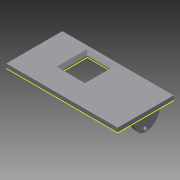
# Autodesk Inventor part: obudowa - timer- back
Saved by Autodesk Inventor 2014 (Build 180170000, 170)
## iProperties
Created: 2018-02-28
Part Number: obudowa - timer- back
Material: Generic
Document SubType Name: Modeling
Designer: HP820
Density: 1 g/cm^3
Appearance: Default
Author: HP820
Autodesk Inventor part; units mm, degrees
ref_plane "YZ Plane" through (0, 0, 0) normal (1, 0, 0) x (0, 1, 0)
ref_plane "XZ Plane" through (0, 0, 0) normal (0, 1, 0) x (-1, 0, 0)
ref_plane "XY Plane" through (0, 0, 0) normal (0, 0, 1) x (1, 0, 0)
sketch "Sketch1" plane through (0, 0, 0) normal (0, 0, 1) x (1, 0, 0)
  line L0 (40, 20.5) -> (40, -20.5) projected
  line L1 (-40, 20.5) -> (40, 20.5) projected
  line L2 (-40, -20.5) -> (-40, 20.5) projected
  line L3 (40, -20.5) -> (-40, -20.5) projected
  line L4 (40, 20.5) -> (40, -20.5) projected
  line L5 (40, -20.5) -> (-40, -20.5) projected
  line L6 (-40, -20.5) -> (-40, 20.5) projected
  line L7 (-40, 20.5) -> (40, 20.5) projected
  line L8 (37, 23.5) -> (-37, 23.5) projected
  line L9 (-43, 17.5) -> (-43, -17.5) projected
  line L10 (-37, -23.5) -> (37, -23.5) projected
  line L11 (43, -17.5) -> (43, 17.5) projected
  line L12 (34.23, -11.25) -> (34.23, 10.75) projected
  line L13 (5.23, -11.25) -> (34.23, -11.25) projected
  line L14 (5.23, 10.75) -> (5.23, -11.25) projected
  line L15 (34.23, 10.75) -> (5.23, 10.75) projected
  circle A0 centre (-26.5, 0.5) radius 5 projected
  arc A1 (37, -23.5) -> (43, -17.5) centre (37, -17.5) ccw projected
  arc A2 (43, 17.5) -> (37, 23.5) centre (37, 17.5) ccw projected
  arc A3 (-37, 23.5) -> (-43, 17.5) centre (-37, 17.5) ccw projected
  arc A4 (-43, -17.5) -> (-37, -23.5) centre (-37, -17.5) ccw projected
  point P0 (0, 0)
extrude "Extrusion1" add sketch "Sketch1" along normal blind 3 contours L0 L3 L2 L1 | A2 L11 A1 L10 A4 L9 A3 L8 | L13 L14 L15 L12 | A0
sketch "Sketch2" plane through (0, 0, 3) normal (0, 0, 1) x (1, 0, 0)
  line L0 (39.5, 20) -> (-39.5, 20) projected
  line L1 (-39.5, 20) -> (-39.5, -20) projected
  line L2 (-39.5, -20) -> (39.5, -20) projected
  line L3 (39.5, -20) -> (39.5, 20) projected
  line L4 (-17.5, 15.5) -> (-1.5, 15.5)
  line L5 (-1.5, 15.5) -> (-1.5, -2)
  line L6 (-1.5, -2) -> (-17.5, -2)
  line L7 (-17.5, -2) -> (-17.5, 15.5)
  line L8 (-17.5, 15.5) -> (-1.5, -2) construction
  line L9 (-1.5, 15.5) -> (-17.5, -2) construction
  point P0 (0, 0)
  point P1 (-9.5, 6.75)
  dimension "d2" = 16
  dimension "d3" = 17.5
  dimension "d4" = 18
  dimension "d6" = 41
  constraints: 12 end point, 2 midpoint, 2 parallel, 1 horizontal, 1 perpendicular
  measures "d2" distance of L5.end L6.end
  measures "d3" distance of L4.end L5.end
  measures "d4" distance between parallel lines of L2 L6
  measures "d6" distance between parallel lines of L3 L5
extrude "Extrusion2" cut sketch "Sketch2" against normal blind 3 contours L4 L5 L6 L7
chamfer "Chamfer1" distance 2 angle 45 4 edges at (-1.5, 6.75, 3) (-17.5, 6.75, 3) (-9.5, -2, 3) (-9.5, 15.5, 3)
sketch "Sketch3" plane through (0, 0, 3) normal (0, 0, 1) x (1, 0, 0)
  line L0 (37, 23.5) -> (-37, 23.5) projected
  arc A0 (-37, 23.5) -> (-43, 17.5) centre (-37, 17.5) ccw projected
  line L1 (-43, 17.5) -> (-43, -17.5) projected
  arc A1 (-43, -17.5) -> (-37, -23.5) centre (-37, -17.5) ccw projected
  line L2 (-37, -23.5) -> (37, -23.5) projected
  arc A2 (37, -23.5) -> (43, -17.5) centre (37, -17.5) ccw projected
  line L3 (43, -17.5) -> (43, 17.5) projected
  arc A3 (43, 17.5) -> (37, 23.5) centre (37, 17.5) ccw projected
  line L4 (34.23, -11.25) -> (34.23, 10.75) projected
  line L5 (5.23, -11.25) -> (34.23, -11.25) projected
  line L6 (5.23, 10.75) -> (5.23, -11.25) projected
  line L7 (34.23, 10.75) -> (5.23, 10.75) projected
  line L8 (40, 20.5) -> (40, -20.5) projected
  line L9 (-40, 20.5) -> (40, 20.5) projected
  line L10 (-40, -20.5) -> (-40, 20.5) projected
  line L11 (40, -20.5) -> (-40, -20.5) projected
  circle A4 centre (-26.5, 0.5) radius 5 projected
  point P0 (0, 0)
extrude "Extrusion3" cut sketch "Sketch3" against normal blind 3 contours A3 L3 A2 L2 A1 L1 A0 L0
sketch "Sketch4" plane through (0, 0, 3) normal (0, 0, 1) x (1, 0, 0)
  line L0 (40, 20.5) -> (-40, 20.5) projected
  line L1 (-40, 20.5) -> (-40, -20.5) projected
  line L2 (-40, -20.5) -> (40, -20.5) projected
  line L3 (40, -20.5) -> (40, 20.5) projected
  line L4 (-39.25, 19.75) -> (39.25, 19.75)
  line L5 (39.25, 19.75) -> (39.25, -19.75)
  line L6 (39.25, -19.75) -> (-39.25, -19.75)
  line L7 (-39.25, -19.75) -> (-39.25, 19.75)
  line L8 (-39.25, 19.75) -> (39.25, -19.75) construction
  line L9 (39.25, 19.75) -> (-39.25, -19.75) construction
  point P0 (0, 0)
  dimension "d14" = 78.5
  dimension "d15" = 39.5
  constraints: 12 end point, 2 midpoint, 2 parallel, 1 horizontal, 1 perpendicular
  measures "d14" distance of L5.end L6.end
  measures "d15" distance of L4.end L5.end
extrude "Extrusion4" cut sketch "Sketch4" against normal blind 3
sketch "Sketch5" plane through (0, 0, 0) normal (0, 0, -1) x (-1, 0, 0)
  line L0 (39.25, -19.75) -> (39.25, 19.75) projected
  line L1 (39.25, 19.75) -> (-39.25, 19.75) projected
  line L2 (-39.25, 19.75) -> (-39.25, -19.75) projected
  line L3 (-39.25, -19.75) -> (39.25, -19.75) projected
  line L4 (17.5, 15.5) -> (17.5, -2) projected
  line L5 (17.5, -2) -> (1.5, -2) projected
  line L6 (1.5, -2) -> (1.5, 15.5) projected
  line L7 (1.5, 15.5) -> (17.5, 15.5) projected
  point P0 (0, 0)
sketch "Sketch6" plane through (39.25, -19.75, 3) normal (1, 0, 0) x (0, 0, -1)
  line L0 (3, 39.5) -> (3, 0) projected
  line L1 (3, 30.3376) -> (7.1898, 28.4353) construction
  line L2 (7.1898, 28.4353) -> (10.8762, 26.1607) construction
  line L3 (10.8762, 26.1607) -> (12.9155, 21.0624) construction
  line L4 (12.9155, 21.0624) -> (12.9155, 15.718) construction
  line L5 (12.9155, 15.718) -> (7.6212, 12.5523) construction
  line L6 (7.6212, 12.5523) -> (3, 10.7087) construction
  spline S0 degree 4 poles (3, 30.3376) (7.1898, 28.4353) (10.8762, 26.1607) (12.9155, 21.0624) (12.9155, 15.718) (7.6212, 12.5523) (3, 10.7087) knots 1 1 1 1 1 2 3 4 4 4 4 4
  line L7 (3, 30.3376) -> (3, 10.7087)
  point P0 (3, 19.75)
  constraints: 2 end point, 2 parallel, 2 point on line, 3 other
extrude "Extrusion5" add sketch "Sketch6" against normal blind 3
sketch "Sketch7" plane through (-39.25, -19.75, 3) normal (-1, 0, 0) x (0, 0, 1)
  line L0 (-3, 30.3376) -> (-3, 10.7087) projected
  spline S0 degree 4 poles (-3, 30.3376) (-7.1898, 28.4353) (-10.8762, 26.1607) (-12.9155, 21.0624) (-12.9155, 15.718) (-7.6212, 12.5523) (-3, 10.7087) knots 0 0 0 0 0 0.333333 0.666667 1 1 1 1 1 projected
  point P0 (-3, 19.75)
  constraints: 1 vertical alignment
extrude "Extrusion6" add sketch "Sketch7" against normal blind 3
sketch "Sketch8" plane through (39.25, -19.75, 3) normal (1, 0, 0) x (0, 0, -1)
  line L0 (0, 0) -> (0, 39.5) projected
  circle A0 centre (10, 19.75) radius 1.2
  point P0 (3, 19.75)
  dimension "d22" = 2.4
  dimension "d23" = 10
  constraints: 1 centre point
  measures "d22" diameter of A0
  measures "d23" distance from line of A0.centre L0
extrude "Extrusion7" cut sketch "Sketch8" against normal through all
chamfer "Chamfer2" distance 0.5 angle 45 2 edges at (39.25, 0, -5.8) (-39.25, 0, -5.8)
sketch "Sketch9" plane through (0, 0, 0) normal (0, 0, -1) x (-1, 0, 0)
  line L0 (39.25, -9.0413) -> (36.25, -9.0413) projected
  line L1 (36.25, -9.0413) -> (36.25, 10.5876) projected
  line L2 (36.25, 10.5876) -> (39.25, 10.5876) projected
  line L3 (39.25, 10.5876) -> (39.25, 19.75) projected
  line L4 (39.25, 19.75) -> (-39.25, 19.75) projected
  line L5 (-39.25, 19.75) -> (-39.25, 10.5876) projected
  line L6 (-39.25, 10.5876) -> (-36.25, 10.5876) projected
  line L7 (-36.25, 10.5876) -> (-36.25, -9.0413) projected
  line L8 (-36.25, -9.0413) -> (-39.25, -9.0413) projected
  line L9 (-39.25, -9.0413) -> (-39.25, -19.75) projected
  line L10 (-39.25, -19.75) -> (39.25, -19.75) projected
  line L11 (39.25, -19.75) -> (39.25, -9.0413) projected
  line L12 (17.5, 15.5) -> (17.5, -2) projected
  line L13 (17.5, -2) -> (1.5, -2) projected
  line L14 (1.5, -2) -> (1.5, 15.5) projected
  line L15 (1.5, 15.5) -> (17.5, 15.5) projected
  point P0 (0, 0)
body "Solid1"
